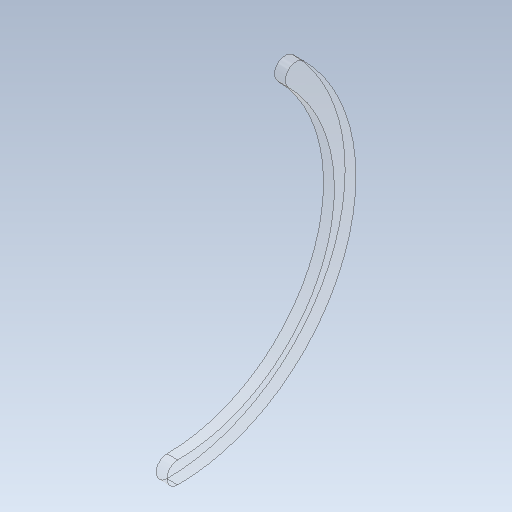
# Autodesk Inventor part: Curved Lexan Support
Saved by Autodesk Inventor 2021 (Build 250183000, 183)
## iProperties
Created: 2021-02-03
Part Number: Curved Lexan Support
Material: Polycarbonate, Clear
Document SubType Name: Modeling
Designer: aidan
Density: 1.2 g/cm^3
Appearance: Polycarbonate - Clear
Author: aidan
Autodesk Inventor part; units mm, degrees
ref_plane "YZ Plane" through (0, 0, 0) normal (1, 0, 0) x (0, 1, 0)
ref_plane "XZ Plane" through (0, 0, 0) normal (0, 1, 0) x (-1, 0, 0)
ref_plane "XY Plane" through (0, 0, 0) normal (0, 0, 1) x (1, 0, 0)
sketch "Sketch1" plane through (0, 0, 0) normal (1, 0, 0) x (0, 1, 0)
  arc A0 (-196.85, 0) -> (139.194, -139.194) centre (0, 0) ccw construction
  arc A1 (-209.55, 0) -> (148.1742, -148.1742) centre (0, 0) ccw
  arc A2 (-184.15, 0) -> (130.2137, -130.2137) centre (0, 0) ccw
  arc A3 (-184.15, 0) -> (-209.55, 0) centre (-196.85, 0) ccw
  arc A4 (148.1742, -148.1742) -> (130.2137, -130.2137) centre (139.194, -139.194) ccw
  line L0 (0, 0) -> (-28.2528, 0) construction
  line L1 (-28.2528, 0) -> (-28.2528, -35.2546) construction
  line L2 (-28.2528, -35.2546) -> (0, -35.2546) construction
  line L3 (0, -35.2546) -> (0, 0) construction
  line L4 (0, 0) -> (258.9139, -258.9139) construction
  dimension "d1" = 45
  dimension "d5" = 209.55
  dimension "d6" = 12.7
  dimension "d7" = 196.85
  dimension "d8" = 184.15
  dimension "d9" = 12.7
  constraints: 10 end point, 10 point on circle, 5 centre point, 4 tangent, 2 parallel, 2 point on line, 1 coincident, 1 horizontal, 1 perpendicular
  measures "d1" angle of L4 L3
  measures "d5" radius of A1
  measures "d6" radial gap between concentric circles of A1 A0
  measures "d7" radius of A0
  measures "d8" radius of A2
  measures "d9" radius of A4
extrude "Extrusion1" add sketch "Sketch1" along normal blind 12.7
body "Solid1"
